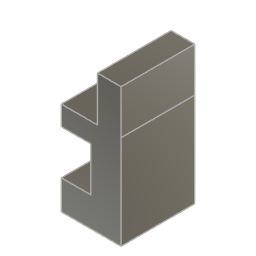
End_cap v3 (Autodesk Fusion 360 design; units mm, degrees)
Autodesk Fusion 360 part; units mm, degrees
sketch "Sketch3" plane through (0, 0, 0) normal (0, 1, 0) x (1, 0, 0)
  line L0 (0, 0) -> (-77.216, 0)
  line L1 (-77.216, 0) -> (-77.216, -38.1)
  line L2 (-77.216, -38.1) -> (-39.116, -38.1)
  line L3 (-39.116, -38.1) -> (-39.116, -95.25)
  line L4 (-39.116, -95.25) -> (-77.216, -95.25)
  line L5 (-77.216, -95.25) -> (-77.216, -120.65)
  line L6 (-77.216, -120.65) -> (-30.4714, -120.65)
  line L7 (-0.0056, -121.5825) -> (0, 0)
  line L8 (-30.4714, -120.65) -> (-30.4714, -178.7325)
  line L9 (-30.4714, -178.7325) -> (-0.0056, -178.7325)
  line L10 (-0.0056, -178.7325) -> (-0.0056, -121.5825)
  dimension "d9" = 77.216
  dimension "d10" = 38.1
  dimension "d11" = 38.1
  dimension "d12" = 57.15
  dimension "d13" = 38.1
  dimension "d14" = 25.4
  dimension "d15" = 77.216
  dimension "d17" = 57.15
  constraint coincident L0.start L7.end
  constraint horizontal L0
  constraint perpendicular L0 L1
  constraint perpendicular L1 L2
  constraint perpendicular L2 L3
  constraint perpendicular L3 L4
  constraint perpendicular L4 L5
  constraint perpendicular L5 L6
  constraint vertical L8
  constraint horizontal L9
  constraint vertical L10
  measures "d9" distance of L0.start L0.end
  measures "d10" distance of L0.end L1.end
  measures "d11" distance of L1.end L2.end
  measures "d12" distance of L2.end L3.end
  measures "d13" distance of L3.end L4.end
  measures "d14" distance of L4.end L5.end
  measures "d15" distance of L5.end L7.start
  measures "d17" distance of L7.start L9.end
extrude "Extrude2" add sketch "Sketch3" along normal blind 95.25
